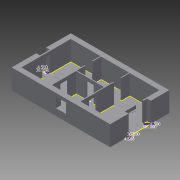
# Autodesk Inventor part: East_Structure
Saved by Autodesk Inventor 2014 (Build 180170000, 170)
## iProperties
Created: 2014-07-16
Part Number: East_Structure
Material: Generic
Document SubType Name: Modeling
Designer: jmw3
Density: 1 g/cm^3
Appearance: Default
Author: jmw3
Autodesk Inventor part; units mm, degrees
ref_plane "YZ Plane" through (0, 0, 0) normal (1, 0, 0) x (0, 1, 0)
ref_plane "XZ Plane" through (0, 0, 0) normal (0, 1, 0) x (-1, 0, 0)
ref_plane "XY Plane" through (0, 0, 0) normal (0, 0, 1) x (1, 0, 0)
sketch "Sketch1" plane through (0, 0, 0) normal (0, 1, 0) x (-1, 0, 0)
  line L0 (3657.6, -6096) -> (3657.6, 6096)
  line L1 (-3657.6, 6096) -> (-3657.6, -6096)
  line L2 (-5120.64, 0) -> (5120.64, 0) projected
  line L3 (0, -32361.8278) -> (0, 33209.6743) projected
  line L4 (-3048, 1714.5) -> (-3048, -1714.5)
  line L5 (3048, -5486.4) -> (3048, -1828.8)
  line L6 (3048, -1714.5) -> (3048, 1714.5)
  line L7 (3048, 1828.8) -> (3048, 5486.4)
  line L8 (-3048, -1828.8) -> (-3048, -5486.4)
  line L9 (-3048, 5486.4) -> (-3048, 1828.8)
  line L10 (-3048, 1714.5) -> (-3048, -1714.5)
  line L11 (-2009.775, -1828.8) -> (-2009.775, -1714.5)
  line L12 (-1095.375, -1828.8) -> (-1095.375, -1714.5)
  line L13 (-3048, -1714.5) -> (-2009.775, -1714.5)
  line L14 (-1095.375, -1714.5) -> (-57.15, -1714.5)
  line L15 (-3048, -1828.8) -> (-2009.775, -1828.8)
  line L16 (2009.775, -1828.8) -> (2009.775, -1714.5)
  line L17 (1095.375, -1828.8) -> (1095.375, -1714.5)
  line L18 (3048, -1714.5) -> (2009.775, -1714.5)
  line L19 (1095.375, -1714.5) -> (57.15, -1714.5)
  line L20 (3048, -1828.8) -> (2009.775, -1828.8)
  line L21 (1095.375, -1828.8) -> (-1095.375, -1828.8)
  line L22 (-2009.775, -1828.8) -> (-3048, -1828.8)
  line L23 (-1095.375, -1828.8) -> (1095.375, -1828.8)
  line L24 (2009.775, -1828.8) -> (3048, -1828.8)
  line L25 (57.15, -1714.5) -> (1095.375, -1714.5)
  line L26 (2009.775, -1714.5) -> (3048, -1714.5)
  line L27 (-2009.775, 1828.8) -> (-2009.775, 1714.5)
  line L28 (-1095.375, 1828.8) -> (-1095.375, 1714.5)
  line L29 (-3048, 1714.5) -> (-2009.775, 1714.5)
  line L30 (-1095.375, 1714.5) -> (-57.15, 1714.5)
  line L31 (-3048, 1828.8) -> (-2009.775, 1828.8)
  line L32 (3048, 1714.5) -> (2009.775, 1714.5)
  line L33 (3048, 1828.8) -> (2009.775, 1828.8)
  line L34 (2009.775, 1828.8) -> (2009.775, 1714.5)
  line L35 (1095.375, 1828.8) -> (1095.375, 1714.5)
  line L36 (1095.375, 1714.5) -> (57.15, 1714.5)
  line L37 (1095.375, 1828.8) -> (-1095.375, 1828.8)
  line L38 (-2009.775, 1828.8) -> (-3048, 1828.8)
  line L39 (-1095.375, 1828.8) -> (1095.375, 1828.8)
  line L40 (2009.775, 1828.8) -> (3048, 1828.8)
  line L41 (57.15, 1714.5) -> (1095.375, 1714.5)
  line L42 (2009.775, 1714.5) -> (3048, 1714.5)
  line L43 (-57.15, -457.2) -> (57.15, -457.2)
  line L44 (57.15, 457.2) -> (-57.15, 457.2)
  line L45 (-457.2, -6096) -> (-457.2, -5486.4)
  line L46 (457.2, -6096) -> (457.2, -5486.4)
  line L47 (-3048, -5486.4) -> (-457.2, -5486.4)
  line L48 (457.2, -5486.4) -> (3048, -5486.4)
  line L49 (-3657.6, -6096) -> (-457.2, -6096)
  line L50 (457.2, -6096) -> (3657.6, -6096)
  line L51 (914.4, 5486.4) -> (914.4, 6096)
  line L52 (-914.4, 6096) -> (-914.4, 5486.4)
  line L53 (3048, 5486.4) -> (914.4, 5486.4)
  line L54 (-914.4, 5486.4) -> (-3048, 5486.4)
  line L55 (3657.6, 6096) -> (914.4, 6096)
  line L56 (-914.4, 6096) -> (-3657.6, 6096)
  line L57 (-57.15, -1714.5) -> (-57.15, -457.2)
  line L58 (-57.15, 457.2) -> (-57.15, 1714.5)
  line L59 (-57.15, 1714.5) -> (-57.15, 457.2)
  line L60 (-57.15, -457.2) -> (-57.15, -1714.5)
  line L61 (57.15, -1714.5) -> (57.15, -457.2)
  line L62 (57.15, 457.2) -> (57.15, 1714.5)
  line L63 (57.15, 1714.5) -> (57.15, 457.2)
  line L64 (57.15, -457.2) -> (57.15, -1714.5)
  line L65 (-3048, 5486.4) -> (-3048, 1828.8)
  line L66 (-3048, 1828.8) -> (-2009.775, 1828.8)
  line L67 (-2009.775, 1828.8) -> (-2009.775, 1714.5)
  line L68 (-2009.775, 1714.5) -> (-3048, 1714.5)
  line L69 (-3048, 1714.5) -> (-3048, -1714.5)
  line L70 (-3048, -1714.5) -> (-2009.775, -1714.5)
  line L71 (-2009.775, -1714.5) -> (-2009.775, -1828.8)
  line L72 (-2009.775, -1828.8) -> (-3048, -1828.8)
  line L73 (-3048, -1828.8) -> (-3048, -5486.4)
  line L74 (-3048, -5486.4) -> (-457.2, -5486.4)
  line L75 (457.2, -5486.4) -> (3048, -5486.4)
  line L76 (3048, -5486.4) -> (3048, -1828.8)
  line L77 (3048, -1828.8) -> (2009.775, -1828.8)
  line L78 (2009.775, -1828.8) -> (2009.775, -1714.5)
  line L79 (2009.775, -1714.5) -> (3048, -1714.5)
  line L80 (3048, 1714.5) -> (3048, -1714.5)
  line L81 (3048, 1714.5) -> (2009.775, 1714.5)
  line L82 (2009.775, 1714.5) -> (2009.775, 1828.8)
  line L83 (2009.775, 1828.8) -> (3048, 1828.8)
  line L84 (3048, 1828.8) -> (3048, 5486.4)
  point P0 (0, 0)
  point P1 (0, 32361.8278)
  point P2 (0, -33209.6743)
  dimension "d2" = 7315.2
  dimension "d10" = 609.6
  dimension "d13" = 1038.225
  dimension "d14" = 914.4
  dimension "d17" = 114.3
  dimension "d18" = 1038.225
  dimension "d19" = 1038.225
  dimension "d20" = 914.4
  dimension "d21" = 914.4
  dimension "d23" = 609.6
  dimension "d24" = 4267.2
  dimension "d25" = 1828.8
  dimension "d26" = 12192
  dimension "d27" = 609.6
  dimension "d28" = 114.3
  constraints: 166 end point, 46 perpendicular, 24 collinear, 24 symmetric about line, 23 parallel, 7 horizontal, 8 other
  measures "d2" distance between parallel lines of L0 L1
  measures "d10" distance between parallel lines of L0 L5
  measures "d13" distance between parallel lines of L10 L11
  measures "d14" distance between parallel lines of L11 L12
  measures "d17" distance between parallel lines of L23 L19
  measures "d18" distance of L4.start L29.end
  measures "d19" distance of L6.end L32.end
  measures "d20" distance between parallel lines of L43 L44
  measures "d21" distance between parallel lines of L46 L45
  measures "d23" distance between parallel lines of L49 L47
  measures "d24" distance between parallel lines of L15 L49
  measures "d25" distance between parallel lines of L51 L52
  measures "d26" distance between parallel lines of L50 L55
  measures "d27" distance between parallel lines of L56 L54
  measures "d28" distance between parallel lines of L64 L57
extrude "Extrusion1" add sketch "Sketch1" along normal blind 2438.4
sketch "Sketch2" plane through (-3657.6, 0, -6096) normal (-1, 0, 0) x (0, 0, 1)
  line L0 (0, 0) -> (12192, 0) projected
  line L1 (5486.4, 2032) -> (6705.6, 2032)
  line L2 (6705.6, 2032) -> (6705.6, 812.8)
  line L3 (6705.6, 812.8) -> (5486.4, 812.8)
  line L4 (5486.4, 812.8) -> (5486.4, 2032)
  line L5 (6096, 2926.08) -> (6096, -487.68) projected
  point P0 (6096, 0)
  dimension "d31" = 1219.2
  dimension "d33" = 1219.2
  dimension "d34" = 812.8
  constraints: 8 end point, 2 parallel, 1 horizontal, 1 perpendicular, 1 other
  measures "d31" distance between parallel lines of L2 L4
  measures "d33" distance between parallel lines of L1 L3
  measures "d34" distance between parallel lines of L0 L3
extrude "Extrusion2" cut sketch "Sketch2" against normal up to surface (609.6 mm away)
sketch "Sketch3" plane through (0, 2438.4, 0) normal (0, 1, 0) x (1, 0, 0)
  line L0 (57.15, 1714.5) -> (1095.375, 1714.5) projected
  line L1 (1095.375, 1714.5) -> (1095.375, 1828.8) projected
  line L2 (1095.375, 1828.8) -> (-1095.375, 1828.8) projected
  line L3 (-1095.375, 1828.8) -> (-1095.375, 1714.5) projected
  line L4 (-1095.375, 1714.5) -> (-57.15, 1714.5) projected
  line L5 (-57.15, 1714.5) -> (-57.15, 457.2) projected
  line L6 (-57.15, 457.2) -> (57.15, 457.2) projected
  line L7 (57.15, 457.2) -> (57.15, 1714.5) projected
  line L8 (-57.15, -1714.5) -> (-1095.375, -1714.5) projected
  line L9 (-1095.375, -1714.5) -> (-1095.375, -1828.8) projected
  line L10 (-1095.375, -1828.8) -> (1095.375, -1828.8) projected
  line L11 (1095.375, -1828.8) -> (1095.375, -1714.5) projected
  line L12 (1095.375, -1714.5) -> (57.15, -1714.5) projected
  line L13 (57.15, -1714.5) -> (57.15, -457.2) projected
  line L14 (57.15, -457.2) -> (-57.15, -457.2) projected
  line L15 (-57.15, -457.2) -> (-57.15, -1714.5) projected
  line L16 (3657.6, 6096) -> (457.2, 6096) projected
  line L17 (457.2, 6096) -> (457.2, 5486.4) projected
  line L18 (457.2, 5486.4) -> (3048, 5486.4) projected
  line L19 (3048, 5486.4) -> (3048, 1828.8) projected
  line L20 (3048, 1828.8) -> (2009.775, 1828.8) projected
  line L21 (2009.775, 1828.8) -> (2009.775, 1714.5) projected
  line L22 (2009.775, 1714.5) -> (3048, 1714.5) projected
  line L23 (3048, 1714.5) -> (3048, -1714.5) projected
  line L24 (3048, -1714.5) -> (2009.775, -1714.5) projected
  line L25 (2009.775, -1714.5) -> (2009.775, -1828.8) projected
  line L26 (2009.775, -1828.8) -> (3048, -1828.8) projected
  line L27 (3048, -1828.8) -> (3048, -5486.4) projected
  line L28 (3048, -5486.4) -> (914.4, -5486.4) projected
  line L29 (914.4, -5486.4) -> (914.4, -6096) projected
  line L30 (914.4, -6096) -> (3657.6, -6096) projected
  line L31 (3657.6, -6096) -> (3657.6, 6096) projected
  line L32 (-457.2, 6096) -> (457.2, 6096)
  line L33 (457.2, 6096) -> (457.2, 5486.4)
  line L34 (457.2, 5486.4) -> (-457.2, 5486.4)
  line L35 (-457.2, 5486.4) -> (-457.2, 6096)
  line L36 (-2009.775, 1828.8) -> (-1095.375, 1828.8)
  line L37 (-1095.375, 1828.8) -> (-1095.375, 1714.5)
  line L38 (-1095.375, 1714.5) -> (-2009.775, 1714.5)
  line L39 (-2009.775, 1714.5) -> (-2009.775, 1828.8)
  line L40 (1095.375, 1828.8) -> (2009.775, 1828.8)
  line L41 (2009.775, 1828.8) -> (2009.775, 1714.5)
  line L42 (2009.775, 1714.5) -> (1095.375, 1714.5)
  line L43 (1095.375, 1714.5) -> (1095.375, 1828.8)
  line L44 (-57.15, 457.2) -> (57.15, 457.2)
  line L45 (57.15, 457.2) -> (57.15, -457.2)
  line L46 (57.15, -457.2) -> (-57.15, -457.2)
  line L47 (-57.15, -457.2) -> (-57.15, 457.2)
  line L48 (1095.375, -1714.5) -> (2009.775, -1714.5)
  line L49 (2009.775, -1714.5) -> (2009.775, -1828.8)
  line L50 (2009.775, -1828.8) -> (1095.375, -1828.8)
  line L51 (1095.375, -1828.8) -> (1095.375, -1714.5)
  line L52 (-2009.775, -1714.5) -> (-1095.375, -1714.5)
  line L53 (-1095.375, -1714.5) -> (-1095.375, -1828.8)
  line L54 (-1095.375, -1828.8) -> (-2009.775, -1828.8)
  line L55 (-2009.775, -1828.8) -> (-2009.775, -1714.5)
  line L56 (-914.4, -5486.4) -> (914.4, -5486.4)
  line L57 (914.4, -5486.4) -> (914.4, -6096)
  line L58 (914.4, -6096) -> (-914.4, -6096)
  line L59 (-914.4, -6096) -> (-914.4, -5486.4)
  line L60 (1095.375, 1828.8) -> (2009.775, 1828.8)
  line L61 (2009.775, 1828.8) -> (2009.775, 1714.5)
  line L62 (2009.775, 1714.5) -> (1095.375, 1714.5)
  line L63 (1095.375, 1714.5) -> (1095.375, 1828.8)
  point P0 (0, 0)
  constraints: 64 end point, 16 parallel, 8 horizontal, 8 perpendicular
extrude "Extrusion3" add sketch "Sketch3" against normal blind 406.4 contours L1 L40 L21 L42 | L45 L14 L47 L6 | L3 L38 L39 L36 | L48 L25 L50 L11 | L9 L54 L55 L52 | L34 L35 L32 L17 | L29 L58 L59 L56
sketch "Sketch5" plane through (0, 0, 0) normal (0, -1, 0) x (1, 0, 0)
  line L0 (3657.6, -6096) -> (457.2, -6096) projected
  line L1 (3657.6, 6096) -> (3657.6, -6096) projected
  line L2 (914.4, 6096) -> (3657.6, 6096) projected
  line L3 (914.4, 5486.4) -> (914.4, 6096) projected
  line L4 (3048, 5486.4) -> (914.4, 5486.4) projected
  line L5 (3048, 1828.8) -> (3048, 5486.4) projected
  line L6 (2009.775, 1828.8) -> (3048, 1828.8) projected
  line L7 (2009.775, 1714.5) -> (2009.775, 1828.8) projected
  line L8 (3048, 1714.5) -> (2009.775, 1714.5) projected
  line L9 (3048, -1714.5) -> (3048, 1714.5) projected
  line L10 (2009.775, -1714.5) -> (3048, -1714.5) projected
  line L11 (2009.775, -1828.8) -> (2009.775, -1714.5) projected
  line L12 (3048, -1828.8) -> (2009.775, -1828.8) projected
  line L13 (3048, -5486.4) -> (3048, -1828.8) projected
  line L14 (457.2, -5486.4) -> (3048, -5486.4) projected
  line L15 (457.2, -6096) -> (457.2, -5486.4) projected
  line L16 (-3657.6, 6096) -> (3657.6, 6096)
  line L17 (3657.6, 6096) -> (3657.6, -6096)
  line L18 (3657.6, -6096) -> (-3657.6, -6096)
  line L19 (-3657.6, -6096) -> (-3657.6, 6096)
  point P0 (0, 0)
  constraints: 8 end point, 2 parallel, 1 horizontal, 1 perpendicular
extrude "Extrusion5" add sketch "Sketch5" along normal blind 25.4
sketch "Sketch6" plane through (0, 2438.4, 0) normal (0, 1, 0) x (1, 0, 0)
  line L0 (-3048, 5486.4) -> (3048, 5486.4) projected
  line L1 (3048, -5486.4) -> (-3048, -5486.4) projected
  line L2 (457.2, 5486.4) -> (457.2, 6096) projected
  line L3 (-457.2, 6096) -> (-457.2, 5486.4) projected
  line L4 (-914.4, -6096) -> (-914.4, -5486.4) projected
  line L5 (914.4, -6096) -> (-914.4, -6096) projected
  line L6 (914.4, -5486.4) -> (914.4, -6096) projected
  line L7 (3048, -5486.4) -> (914.4, -5486.4) projected
  line L8 (3048, -1828.8) -> (3048, -5486.4) projected
  line L9 (2009.775, -1828.8) -> (3048, -1828.8) projected
  line L10 (2009.775, -1714.5) -> (2009.775, -1828.8) projected
  line L11 (3048, -1714.5) -> (2009.775, -1714.5) projected
  line L12 (3048, 1714.5) -> (3048, -1714.5) projected
  line L13 (2009.775, 1714.5) -> (3048, 1714.5) projected
  line L14 (2009.775, 1828.8) -> (2009.775, 1714.5) projected
  line L15 (3048, 1828.8) -> (2009.775, 1828.8) projected
  line L16 (3048, 5486.4) -> (3048, 1828.8) projected
  line L17 (457.2, 5486.4) -> (3048, 5486.4) projected
  line L18 (457.2, 6096) -> (457.2, 5486.4) projected
  line L19 (-457.2, 6096) -> (457.2, 6096) projected
  line L20 (-457.2, 5486.4) -> (-457.2, 6096) projected
  line L21 (-3048, 5486.4) -> (-457.2, 5486.4) projected
  line L22 (-3048, 1828.8) -> (-3048, 5486.4) projected
  line L23 (-2009.775, 1828.8) -> (-3048, 1828.8) projected
  line L24 (-2009.775, 1714.5) -> (-2009.775, 1828.8) projected
  line L25 (-3048, 1714.5) -> (-2009.775, 1714.5) projected
  line L26 (-3048, -1714.5) -> (-3048, 1714.5) projected
  line L27 (-2009.775, -1714.5) -> (-3048, -1714.5) projected
  line L28 (-2009.775, -1828.8) -> (-2009.775, -1714.5) projected
  line L29 (-3048, -1828.8) -> (-2009.775, -1828.8) projected
  line L30 (-3048, -5486.4) -> (-3048, -1828.8) projected
  line L31 (-914.4, -5486.4) -> (-3048, -5486.4) projected
  line L32 (1095.375, -1714.5) -> (57.15, -1714.5) projected
  line L33 (1095.375, -1828.8) -> (1095.375, -1714.5) projected
  line L34 (-1095.375, -1828.8) -> (1095.375, -1828.8) projected
  line L35 (-1095.375, -1714.5) -> (-1095.375, -1828.8) projected
  line L36 (-57.15, -1714.5) -> (-1095.375, -1714.5) projected
  line L37 (-57.15, -457.2) -> (-57.15, -1714.5) projected
  line L38 (57.15, -457.2) -> (-57.15, -457.2) projected
  line L39 (57.15, -1714.5) -> (57.15, -457.2) projected
  line L40 (-57.15, 457.2) -> (57.15, 457.2) projected
  line L41 (-57.15, 1714.5) -> (-57.15, 457.2) projected
  line L42 (-1095.375, 1714.5) -> (-57.15, 1714.5) projected
  line L43 (-1095.375, 1828.8) -> (-1095.375, 1714.5) projected
  line L44 (1095.375, 1828.8) -> (-1095.375, 1828.8) projected
  line L45 (1095.375, 1714.5) -> (1095.375, 1828.8) projected
  line L46 (57.15, 1714.5) -> (1095.375, 1714.5) projected
  line L47 (57.15, 457.2) -> (57.15, 1714.5) projected
  line L48 (-457.2, 6096) -> (457.2, 6096)
  line L49 (457.2, 6096) -> (457.2, 5638.8)
  line L50 (457.2, 5638.8) -> (-457.2, 5638.8)
  line L51 (-457.2, 5638.8) -> (-457.2, 6096)
  line L52 (-914.4, -6096) -> (914.4, -6096)
  line L53 (914.4, -6096) -> (914.4, -5638.8)
  line L54 (914.4, -5638.8) -> (-914.4, -5638.8)
  line L55 (-914.4, -5638.8) -> (-914.4, -6096)
  point P0 (0, 0)
  dimension "d46" = 152.4
  dimension "d47" = 152.4
  constraints: 16 end point, 4 parallel, 2 horizontal, 2 perpendicular, 2 point on line
  measures "d46" distance between parallel lines of L0 L50
  measures "d47" distance between parallel lines of L1 L54
extrude "Extrusion6" cut sketch "Sketch6" against normal up to next contours L3 L19 L2 L50 | L54 L6 L5 L4
sketch "Sketch7" plane through (0, 2438.4, 0) normal (0, 1, 0) x (1, 0, 0)
  line L0 (-914.4, -5638.8) -> (914.4, -5638.8) projected
  line L1 (3048, -5486.4) -> (-3048, -5486.4) projected
  line L2 (0, -5638.8) -> (914.4, -5638.8)
  line L3 (914.4, -5638.8) -> (914.4, -5486.4)
  line L4 (914.4, -5486.4) -> (0, -5486.4)
  line L5 (0, -5486.4) -> (0, -5638.8)
  point P0 (0, 0)
  constraints: 8 end point, 2 parallel, 1 horizontal, 1 midpoint, 1 perpendicular, 1 point on line
extrude "Extrusion7" cut sketch "Sketch7" against normal up to next
sketch "Sketch8" plane through (0, 2438.4, 0) normal (0, 1, 0) x (1, 0, 0)
  line L0 (3657.6, 6096) -> (457.2, 6096) projected
  line L1 (-457.2, 5638.8) -> (-457.2, 6096) projected
  line L2 (-457.2, 6096) -> (-3657.6, 6096) projected
  line L3 (-914.4, -6096) -> (-914.4, -5638.8) projected
  line L4 (-914.4, -5638.8) -> (0, -5638.8) projected
  line L5 (-914.4, -6096) -> (-1371.6, -6096)
  line L6 (-1371.6, -6096) -> (-1371.6, -5638.8)
  line L7 (-1371.6, -5638.8) -> (-914.4, -5638.8)
  line L8 (-914.4, -5638.8) -> (-914.4, -6096)
  line L9 (914.4, -6096) -> (1371.6, -6096)
  line L10 (1371.6, -6096) -> (1371.6, -5638.8)
  line L11 (1371.6, -5638.8) -> (914.4, -5638.8)
  line L12 (914.4, -5638.8) -> (914.4, -6096)
  line L13 (457.2, 5638.8) -> (609.6, 5638.8)
  line L14 (609.6, 5638.8) -> (609.6, 6096)
  line L15 (609.6, 6096) -> (457.2, 6096)
  line L16 (457.2, 6096) -> (457.2, 5638.8)
  line L17 (-457.2, 5638.8) -> (-609.6, 5638.8)
  line L18 (-609.6, 5638.8) -> (-609.6, 6096)
  line L19 (-609.6, 6096) -> (-457.2, 6096)
  line L20 (-457.2, 6096) -> (-457.2, 5638.8)
  point P0 (0, 0)
  dimension "d52" = 457.2
  dimension "d53" = 457.2
  dimension "d54" = 152.4
  dimension "d55" = 152.4
  constraints: 32 end point, 8 parallel, 4 horizontal, 4 perpendicular, 2 collinear, 2 point on line
  measures "d52" distance between parallel lines of L3 L6
  measures "d53" distance between parallel lines of L12 L10
  measures "d54" distance between parallel lines of L16 L14
  measures "d55" distance between parallel lines of L20 L18
extrude "Extrusion8" cut sketch "Sketch8" against normal up to surface (2438.4 mm away)
sketch "Sketch9" plane through (0, 2438.4, 0) normal (0, 1, 0) x (1, 0, 0)
  line L0 (1095.375, -1714.5) -> (57.15, -1714.5) projected
  line L1 (1095.375, -1828.8) -> (1095.375, -1714.5) projected
  line L2 (-1095.375, -1828.8) -> (1095.375, -1828.8) projected
  line L3 (-1095.375, -1714.5) -> (-1095.375, -1828.8) projected
  line L4 (-57.15, -1714.5) -> (-1095.375, -1714.5) projected
  line L5 (-57.15, -457.2) -> (-57.15, -1714.5) projected
  line L6 (57.15, -457.2) -> (-57.15, -457.2) projected
  line L7 (57.15, -1714.5) -> (57.15, -457.2) projected
  line L8 (-57.15, 457.2) -> (57.15, 457.2) projected
  line L9 (-57.15, 1714.5) -> (-57.15, 457.2) projected
  line L10 (-1095.375, 1714.5) -> (-57.15, 1714.5) projected
  line L11 (-1095.375, 1828.8) -> (-1095.375, 1714.5) projected
  line L12 (1095.375, 1828.8) -> (-1095.375, 1828.8) projected
  line L13 (1095.375, 1714.5) -> (1095.375, 1828.8) projected
  line L14 (57.15, 1714.5) -> (1095.375, 1714.5) projected
  line L15 (57.15, 457.2) -> (57.15, 1714.5) projected
  line L16 (914.4, -5486.4) -> (914.4, -5638.8) projected
  line L17 (3048, -5486.4) -> (914.4, -5486.4) projected
  line L18 (3048, -1828.8) -> (3048, -5486.4) projected
  line L19 (2009.775, -1828.8) -> (3048, -1828.8) projected
  line L20 (2009.775, -1714.5) -> (2009.775, -1828.8) projected
  line L21 (3048, -1714.5) -> (2009.775, -1714.5) projected
  line L22 (3048, 1714.5) -> (3048, -1714.5) projected
  line L23 (2009.775, 1714.5) -> (3048, 1714.5) projected
  line L24 (2009.775, 1828.8) -> (2009.775, 1714.5) projected
  line L25 (3048, 1828.8) -> (2009.775, 1828.8) projected
  line L26 (3048, 5486.4) -> (3048, 1828.8) projected
  line L27 (457.2, 5486.4) -> (3048, 5486.4) projected
  line L28 (457.2, 5638.8) -> (457.2, 5486.4) projected
  line L29 (609.6, 5638.8) -> (457.2, 5638.8) projected
  line L30 (609.6, 6096) -> (609.6, 5638.8) projected
  line L31 (-609.6, 6096) -> (609.6, 6096) projected
  line L32 (-609.6, 5638.8) -> (-609.6, 6096) projected
  line L33 (-457.2, 5638.8) -> (-609.6, 5638.8) projected
  line L34 (-457.2, 5486.4) -> (-457.2, 5638.8) projected
  line L35 (-3048, 5486.4) -> (-457.2, 5486.4) projected
  line L36 (-3048, 1828.8) -> (-3048, 5486.4) projected
  line L37 (-2009.775, 1828.8) -> (-3048, 1828.8) projected
  line L38 (-2009.775, 1714.5) -> (-2009.775, 1828.8) projected
  line L39 (-3048, 1714.5) -> (-2009.775, 1714.5) projected
  line L40 (-3048, -1714.5) -> (-3048, 1714.5) projected
  line L41 (-2009.775, -1714.5) -> (-3048, -1714.5) projected
  line L42 (-2009.775, -1828.8) -> (-2009.775, -1714.5) projected
  line L43 (-3048, -1828.8) -> (-2009.775, -1828.8) projected
  line L44 (-3048, -5486.4) -> (-3048, -1828.8) projected
  line L45 (-914.4, -5486.4) -> (-3048, -5486.4) projected
  line L46 (-914.4, -5638.8) -> (-914.4, -5486.4) projected
  line L47 (-1371.6, -5638.8) -> (-914.4, -5638.8) projected
  line L48 (-1371.6, -6096) -> (-1371.6, -5638.8) projected
  line L49 (1371.6, -6096) -> (-1371.6, -6096) projected
  line L50 (1371.6, -5638.8) -> (1371.6, -6096) projected
  line L51 (914.4, -5638.8) -> (1371.6, -5638.8) projected
  line L52 (1095.375, 1828.8) -> (2009.775, 1828.8)
  line L53 (2009.775, 1828.8) -> (2009.775, 1714.5)
  line L54 (2009.775, 1714.5) -> (1095.375, 1714.5)
  line L55 (1095.375, 1714.5) -> (1095.375, 1828.8)
  line L56 (1095.375, -1714.5) -> (2009.775, -1714.5)
  line L57 (2009.775, -1714.5) -> (2009.775, -1828.8)
  line L58 (2009.775, -1828.8) -> (1095.375, -1828.8)
  line L59 (1095.375, -1828.8) -> (1095.375, -1714.5)
  point P0 (0, 0)
  constraints: 16 end point, 4 parallel, 2 horizontal, 2 perpendicular
extrude "Extrusion9" cut sketch "Sketch9" against normal up to next contours L56 L20 L58 L1 | L54 L13 L52 L24
sketch "Open Doors" plane through (0, 0, 0) normal (0, 1, 0) x (1, 0, 0)
  line L0 (2009.775, -1714.5) -> (2009.775, -1828.8) projected
  line L1 (3048, -1714.5) -> (2009.775, -1714.5) projected
  line L2 (3048, 1714.5) -> (3048, -1714.5) projected
  line L3 (2009.775, 1714.5) -> (3048, 1714.5) projected
  line L4 (2009.775, 1828.8) -> (2009.775, 1714.5) projected
  line L5 (3048, 1828.8) -> (2009.775, 1828.8) projected
  line L6 (3048, 5486.4) -> (3048, 1828.8) projected
  line L7 (457.2, 5486.4) -> (3048, 5486.4) projected
  line L8 (457.2, 5638.8) -> (457.2, 5486.4) projected
  line L9 (609.6, 5638.8) -> (457.2, 5638.8) projected
  line L10 (609.6, 6096) -> (609.6, 5638.8) projected
  line L11 (-609.6, 6096) -> (609.6, 6096) projected
  line L12 (-609.6, 5638.8) -> (-609.6, 6096) projected
  line L13 (-457.2, 5638.8) -> (-609.6, 5638.8) projected
  line L14 (-457.2, 5486.4) -> (-457.2, 5638.8) projected
  line L15 (-3048, 5486.4) -> (-457.2, 5486.4) projected
  line L16 (-3048, 1828.8) -> (-3048, 5486.4) projected
  line L17 (-2009.775, 1828.8) -> (-3048, 1828.8) projected
  line L18 (-2009.775, 1714.5) -> (-2009.775, 1828.8) projected
  line L19 (-3048, 1714.5) -> (-2009.775, 1714.5) projected
  line L20 (-3048, -1714.5) -> (-3048, 1714.5) projected
  line L21 (-2009.775, -1714.5) -> (-3048, -1714.5) projected
  line L22 (-2009.775, -1828.8) -> (-2009.775, -1714.5) projected
  line L23 (-3048, -1828.8) -> (-2009.775, -1828.8) projected
  line L24 (-3048, -5486.4) -> (-3048, -1828.8) projected
  line L25 (-914.4, -5486.4) -> (-3048, -5486.4) projected
  line L26 (-914.4, -5638.8) -> (-914.4, -5486.4) projected
  line L27 (-1371.6, -5638.8) -> (-914.4, -5638.8) projected
  line L28 (-1371.6, -6096) -> (-1371.6, -5638.8) projected
  line L29 (1371.6, -6096) -> (-1371.6, -6096) projected
  line L30 (1371.6, -5638.8) -> (1371.6, -6096) projected
  line L31 (914.4, -5638.8) -> (1371.6, -5638.8) projected
  line L32 (914.4, -5486.4) -> (914.4, -5638.8) projected
  line L33 (3048, -5486.4) -> (914.4, -5486.4) projected
  line L34 (3048, -1828.8) -> (3048, -5486.4) projected
  line L35 (2009.775, -1828.8) -> (3048, -1828.8) projected
  line L36 (57.15, 1714.5) -> (1095.375, 1714.5) projected
  line L37 (57.15, 457.2) -> (57.15, 1714.5) projected
  line L38 (-57.15, 457.2) -> (57.15, 457.2) projected
  line L39 (-57.15, 1714.5) -> (-57.15, 457.2) projected
  line L40 (-1095.375, 1714.5) -> (-57.15, 1714.5) projected
  line L41 (-1095.375, 1828.8) -> (-1095.375, 1714.5) projected
  line L42 (1095.375, 1828.8) -> (-1095.375, 1828.8) projected
  line L43 (1095.375, 1714.5) -> (1095.375, 1828.8) projected
  line L44 (-1095.375, -1828.8) -> (1095.375, -1828.8) projected
  line L45 (-1095.375, -1714.5) -> (-1095.375, -1828.8) projected
  line L46 (-57.15, -1714.5) -> (-1095.375, -1714.5) projected
  line L47 (-57.15, -457.2) -> (-57.15, -1714.5) projected
  line L48 (57.15, -457.2) -> (-57.15, -457.2) projected
  line L49 (57.15, -1714.5) -> (57.15, -457.2) projected
  line L50 (1095.375, -1714.5) -> (57.15, -1714.5) projected
  line L51 (1095.375, -1828.8) -> (1095.375, -1714.5) projected
  line L52 (457.2, 5638.8) -> (746.3587, 6506.276)
  line L53 (746.3587, 6506.276) -> (637.9242, 6542.4208)
  line L54 (637.9242, 6542.4208) -> (348.7655, 5674.9448)
  line L55 (348.7655, 5674.9448) -> (457.2, 5638.8)
  line L56 (914.4, -5638.8) -> (1560.9784, -6285.3784)
  line L57 (1560.9784, -6285.3784) -> (1480.1561, -6366.2007)
  line L58 (1480.1561, -6366.2007) -> (833.5777, -5719.6223)
  line L59 (833.5777, -5719.6223) -> (914.4, -5638.8)
  line L60 (-914.4, -5638.8) -> (-1560.9784, -6285.3784)
  line L61 (-1560.9784, -6285.3784) -> (-1480.1561, -6366.2007)
  line L62 (-1480.1561, -6366.2007) -> (-833.5777, -5719.6223)
  line L63 (-833.5777, -5719.6223) -> (-914.4, -5638.8)
  point P0 (0, 0)
  dimension "d60" = 914.4
  dimension "d62" = 114.3
  dimension "d63" = 914.4
  dimension "d64" = 114.3
  dimension "d65" = 914.4
  dimension "d66" = 114.3
  constraints: 24 end point, 6 parallel, 3 perpendicular, 3 point on line
  measures "d60" distance between parallel lines of L53 L55
  measures "d62" distance between parallel lines of L52 L54
  measures "d63" distance between parallel lines of L59 L57
  measures "d64" distance between parallel lines of L56 L58
  measures "d65" distance between parallel lines of L63 L61
  measures "d66" distance between parallel lines of L60 L62
sketch "Instruments" plane through (0, 0, 0) normal (0, 1, 0) x (1, 0, 0)
  line L0 (3048, 5486.4) -> (3048, 1828.8) projected
  line L1 (457.2, 5486.4) -> (3048, 5486.4) projected
  line L2 (457.2, 5638.8) -> (457.2, 5486.4) projected
  line L3 (-914.4, -5638.8) -> (-914.4, -5486.4) projected
  line L4 (3048, -5486.4) -> (914.4, -5486.4) projected
  line L5 (458.4, 4876.8) -> (2438.4, 4876.8)
  line L6 (2438.4, 4876.8) -> (2438.4, 4216.8)
  line L7 (2438.4, 4216.8) -> (458.4, 4216.8)
  line L8 (458.4, 4216.8) -> (458.4, 4876.8)
  line L9 (0, 9124.1452) -> (0, -8947.9251) projected
  line L10 (-152.4, 5334) -> (-152.4, 5638.8)
  line L11 (-152.4, 5638.8) -> (152.4, 5638.8)
  line L12 (-152.4, 5334) -> (152.4, 5638.8)
  circle A0 centre (-1552.4, 3656) radius 152.4
  circle A1 centre (1547.6, 3656) radius 152.4
  circle A2 centre (1547.6, -4) radius 152.4
  circle A3 centre (-1552.4, -3654) radius 152.4
  circle A4 centre (1547.6, -3654) radius 152.4
  line L13 (-1552.4, 3808.4) -> (-1247.6, 3808.4)
  line L14 (-1247.6, 3808.4) -> (-1247.6, 3503.6)
  line L15 (-1247.6, 3503.6) -> (-1552.4, 3503.6)
  line L16 (-1552.4, 3503.6) -> (-1552.4, 3808.4)
  line L17 (3657.6, 6096) -> (3657.6, -6096) projected
  line L18 (1547.6, 3808.4) -> (1242.8, 3808.4)
  line L19 (1242.8, 3808.4) -> (1242.8, 3503.6)
  line L20 (1242.8, 3503.6) -> (1547.6, 3503.6)
  line L21 (1547.6, 3503.6) -> (1547.6, 3808.4)
  line L22 (-3657.6, 6096) -> (3657.6, 6096) projected
  line L23 (1547.6, 148.4) -> (1242.8, 148.4)
  line L24 (1242.8, 148.4) -> (1242.8, -156.4)
  line L25 (1242.8, -156.4) -> (1547.6, -156.4)
  line L26 (1547.6, -156.4) -> (1547.6, 148.4)
  line L27 (1547.6, -3501.6) -> (1242.8, -3501.6)
  line L28 (1242.8, -3501.6) -> (1242.8, -3806.4)
  line L29 (1242.8, -3806.4) -> (1547.6, -3806.4)
  line L30 (1547.6, -3806.4) -> (1547.6, -3501.6)
  line L31 (-1552.4, 3656) -> (-1640.3882, 3503.6)
  line L32 (-1640.3882, 3503.6) -> (-1816.3645, 3503.6)
  line L33 (-1816.3645, 3503.6) -> (-1904.3527, 3656)
  line L34 (-1904.3527, 3656) -> (-1816.3645, 3808.4)
  line L35 (-1816.3645, 3808.4) -> (-1640.3882, 3808.4)
  line L36 (-1640.3882, 3808.4) -> (-1552.4, 3656)
  line L37 (1547.6, -3654) -> (1635.5882, -3501.6)
  line L38 (1635.5882, -3501.6) -> (1811.5645, -3501.6)
  line L39 (1811.5645, -3501.6) -> (1899.5527, -3654)
  line L40 (1899.5527, -3654) -> (1811.5645, -3806.4)
  line L41 (1811.5645, -3806.4) -> (1635.5882, -3806.4)
  line L42 (1635.5882, -3806.4) -> (1547.6, -3654)
  line L43 (-1552.4, -3501.6) -> (-1247.6, -3501.6)
  line L44 (-1247.6, -3501.6) -> (-1247.6, -3806.4)
  line L45 (-1247.6, -3806.4) -> (-1552.4, -3806.4)
  line L46 (-1552.4, -3806.4) -> (-1552.4, -3501.6)
  line L47 (457.2, -5638.8) -> (458.4, -5638.8)
  line L48 (609.6, -5334) -> (304.8, -5334)
  line L49 (304.8, -5334) -> (304.8, -5638.8)
  line L50 (609.6, -5334) -> (304.8, -5638.8)
  line L51 (-304.8, -5334) -> (-609.6, -5334)
  line L52 (-609.6, -5334) -> (-609.6, -5638.8)
  line L53 (-304.8, -5334) -> (-609.6, -5638.8)
  point P0 (0, 0)
  point P1 (-1728.3764, 3656)
  point P2 (1723.5764, -3654)
  dimension "d83" = 304.8
  dimension "d84" = 304.8
  dimension "d85" = 304.8
  dimension "d86" = 304.8
  dimension "d87" = 304.8
  dimension "d73" = 1980
  dimension "d74" = 660
  dimension "d75" = 609.6
  dimension "d76" = 609.6
  dimension "d79" = 152.4
  dimension "d80" = 152.4
  dimension "d81" = 304.8
  dimension "d82" = 304.8
  dimension "d88" = 304.8
  dimension "d89" = 304.8
  dimension "d91" = 5210
  dimension "d92" = 304.8
  dimension "d93" = 304.8
  dimension "d94" = 2110
  dimension "d95" = 2440
  dimension "d96" = 2440
  dimension "d97" = 2110
  dimension "d98" = 6100
  dimension "d99" = 304.8
  dimension "d100" = 9750
  dimension "d101" = 2110
  dimension "d102" = 304.8
  dimension "d103" = 9750
  dimension "d104" = 5210
  dimension "d108" = 304.8
  dimension "d109" = 304.8
  dimension "d110" = 304.8
  dimension "d111" = 152.4
  dimension "d113" = 304.8
  dimension "d114" = 304.8
  dimension "d115" = 304.8
  constraints: 92 end point, 13 parallel, 10 collinear, 10 horizontal, 7 perpendicular, 5 vertical alignment, 2 point on line, 37 other
  measures "d73" distance between parallel lines of L6 L8
  measures "d74" distance between parallel lines of L5 L7
  measures "d75" distance between parallel lines of L1 L5
  measures "d76" distance between parallel lines of L0 L6
  measures "d79" distance between parallel lines of L1 L11
  measures "d80" distance between parallel lines of L9 L10
  measures "d81" distance of L10.start L10.end
  measures "d82" distance of L10.end L11.end
  measures "d88" distance between parallel lines of L14 L16
  measures "d89" distance between parallel lines of L15 L13
  measures "d91" distance from line of L17 L31.start
  measures "d92" distance between parallel lines of L19 L21
  measures "d93" distance between parallel lines of L20 L18
  measures "d94" distance from line of L17 point (1547.6, 3656)
  measures "d95" distance from line of L22 point (1547.6, 3656)
  measures "d96" distance from line of L22 L31.start
  measures "d97" distance from line of L17 point (1547.6, -4)
  measures "d98" distance from line of L22 point (1547.6, -4)
  measures "d99" distance between parallel lines of L23 L25
  measures "d100" distance from line of L22 L37.start
  measures "d101" distance from line of L17 L37.start
  measures "d102" distance between parallel lines of L27 L29
  measures "d103" distance from line of L22 point (-1552.4, -3654)
  measures "d104" distance from line of L17 point (-1552.4, -3654)
  measures "d108" distance between parallel lines of L9 L49
  measures "d109" distance of L48.start L48.end
  measures "d110" distance of L48.end L49.end
  measures "d111" distance between parallel lines of L4 L48
  measures "d113" distance of L51.end L52.end
  measures "d114" distance of L51.start L51.end
  measures "d115" distance between parallel lines of L3 L52
extrude "Extrusion11" add sketch "Instruments" along normal blind 25.4
sketch "Sketch11" plane through (0, 2438.4, 0) normal (0, 1, 0) x (1, 0, 0)
  line L0 (3657.6, -6096) -> (3657.6, 6096) projected
  line L1 (3657.6, 6096) -> (609.6, 6096) projected
  line L2 (965.2, 406.4) -> (2133.6, 406.4)
  line L3 (2133.6, 406.4) -> (2133.6, -762)
  line L4 (2133.6, -762) -> (965.2, -762)
  line L5 (965.2, -762) -> (965.2, 406.4)
  point P0 (0, 0)
  dimension "d67" = 5689.6
  dimension "d68" = 1524
  dimension "d69" = 1168.4
  dimension "d70" = 1168.4
  constraints: 8 end point, 2 parallel, 1 horizontal, 1 perpendicular
  measures "d67" distance between parallel lines of L1 L2
  measures "d68" distance between parallel lines of L0 L3
  measures "d69" distance between parallel lines of L4 L2
  measures "d70" distance between parallel lines of L3 L5
body "Solid1"
